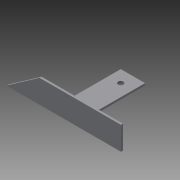
# Autodesk Inventor part: Left Forearm
Saved by Autodesk Inventor 2014 (Build 180170000, 170)
## iProperties
Created: 2015-08-01
Part Number: Left Forearm
Material: Generic
Document SubType Name: Modeling
Designer: Devon
Density: 1 g/cm^3
Appearance: Default
Author: Devon
Autodesk Inventor part; units mm, degrees
ref_plane "YZ Plane" through (0, 0, 0) normal (1, 0, 0) x (0, 1, 0)
ref_plane "XZ Plane" through (0, 0, 0) normal (0, 1, 0) x (-1, 0, 0)
ref_plane "XY Plane" through (0, 0, 0) normal (0, 0, 1) x (1, 0, 0)
sketch "Sketch1" plane through (0, 0, 0) normal (0, 0, 1) x (1, 0, 0)
  line L0 (-26.4763, -7.5222) -> (152.9112, -7.5222)
  line L1 (-26.4763, -7.5222) -> (25.5399, 28.8999)
  line L2 (-26.4763, -7.5222) -> (37.0237, -7.5222) construction
  line L3 (25.5399, 28.8999) -> (152.9112, 28.8999)
  line L4 (152.9112, 28.8999) -> (152.9112, -7.5222)
  point P0 (0, 0)
  dimension "d0" = 179.3875
  dimension "d2" = 63.5
  dimension "d3" = 35
  constraints: 10 end point, 2 horizontal, 1 equal length, 1 perpendicular
  measures "d0" distance of L0.start L0.end
  measures "d2" distance of L0.start L1.end
  measures "d3" angle of L2 L1
extrude "Extrusion1" add sketch "Sketch1" along normal blind 3.175
sketch "Sketch2" plane through (0, 0, 0) normal (0, 0, -1) x (-1, 0, 0)
  line L0 (-152.9112, -7.5222) -> (-152.9112, 28.8999) projected
  line L1 (-152.9112, 28.8999) -> (-25.5399, 28.8999)
  line L2 (-89.2255, 21.9149) -> (-70.1755, 21.9149)
  line L3 (-70.1755, 21.9149) -> (-70.1755, 18.7399)
  line L4 (-70.1755, 18.7399) -> (-108.2755, 18.7399)
  line L5 (-108.2755, 18.7399) -> (-108.2755, 21.9149)
  line L6 (-108.2755, 21.9149) -> (-89.2255, 21.9149)
  point P0 (0, 0)
  dimension "d7" = 19.05
  dimension "d8" = 3.175
  dimension "d9" = 38.1
  dimension "d10" = 3.175
  constraints: 12 end point, 1 parallel, 1 perpendicular
  measures "d7" distance of L2.start L2.end
  measures "d8" distance of L2.end L3.end
  measures "d9" distance of L3.end L4.end
  measures "d10" distance of L4.end L5.end
extrude "Extrusion2" add sketch "Sketch2" along normal blind 79.2734
sketch "Sketch3" plane through (70.1755, 18.7399, 0) normal (0, -1, 0) x (1, 0, 0)
  line L0 (0, -79.2734) -> (19.05, -79.2734)
  line L1 (19.05, -79.2734) -> (19.05, -60.2234)
  line L2 (19.05, -60.2234) -> (0, -60.2234)
  line L3 (0, -60.2234) -> (0, -79.2734)
  point P0 (-70.1755, 0)
  dimension "d13" = 19.05
  dimension "d14" = 19.05
  constraints: 8 end point, 2 parallel, 1 horizontal, 1 perpendicular
  measures "d13" distance of L2.end L1.end
  measures "d14" distance of L1.end L0.end
hole "Hole1" at (89.2255, 18.7399, -60.2234) direction (0, 1, 0) diameter 8.3312 end through all
body "Solid1"
